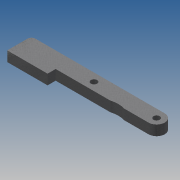
# Autodesk Inventor part: Drückbrücke
Saved by Autodesk Inventor 2015 SP1 (Build 190203100, 203)
## iProperties
Created: 2015-01-28
Part Number: Drückbrücke
Material: ABS-Kunststoff
Document SubType Name: Modeling
Designer: Marc
Density: 1.06 g/cm^3
Appearance: Gehont - dunkelgrau
Mass: 3.36639 g
Surface Area: 19.9083 cm^2
Volume: 3.17584 cm^3
Author: Marc
Autodesk Inventor part; units mm, degrees
ref_plane "YZ Plane" through (0, 0, 0) normal (1, 0, 0) x (0, 1, 0)
ref_plane "XZ Plane" through (0, 0, 0) normal (0, 1, 0) x (-1, 0, 0)
ref_plane "XY Plane" through (0, 0, 0) normal (0, 0, 1) x (1, 0, 0)
sketch "Skizze1" plane through (0, 0, 0) normal (0, 0, 1) x (1, 0, 0)
  line L0 (0, -28.5) -> (0, 27.5) projected
  line L1 (-71.9, 0) -> (35.9, 0) projected
  circle A0 centre (-15.5, 15.5) radius 1.55
  circle A1 centre (15.5, 15.5) radius 1.55
  circle A2 centre (-15.5, -15.5) radius 1.55
  circle A3 centre (15.5, -15.5) radius 1.55
  circle A4 centre (-16.5, 0) radius 11
  circle A5 centre (0, 0) radius 5.5
  circle A6 centre (-16.5, 0) radius 4
  arc A7 (-16.5, -7.5) -> (-16.5, 7.5) centre (-16.5, 0) ccw
  line L2 (-16.5, 7.5) -> (-36.5, 7.5)
  line L3 (-36.5, 7.5) -> (-56.5, 7.5)
  line L4 (-56.5, 7.5) -> (-56.5, -7.5)
  line L5 (-56.5, -7.5) -> (-16.5, -7.5)
  circle A8 centre (15.5, 15.5) radius 4
  circle A9 centre (15.5, -15.5) radius 5
  circle A10 centre (-15.5, 15.5) radius 4
  circle A11 centre (-15.5, -15.5) radius 4
  line L6 (15.5, 11.5) -> (-15.5, 11.5)
  line L7 (15.5, 19.5) -> (-15.5, 19.5)
  line L8 (-15.5, 19.5) -> (-50.5, 19.5)
  line L9 (-50.5, 19.5) -> (-50.5, 7.5)
  line L10 (-15.5, 11.5) -> (-30.5, 11.5)
  line L11 (-30.5, 11.5) -> (-30.5, 7.5)
  dimension "d0" = 3.1
  dimension "d1" = 15.5
  dimension "d2" = 15.5
  dimension "d3" = 22
  dimension "d4" = 16.5
  dimension "d5" = 11
  dimension "d6" = 8
  dimension "d7" = 15
  dimension "d10" = 15
  dimension "d11" = 40
  dimension "d17" = 8
  dimension "d18" = 10
  dimension "d19" = 8
  dimension "d20" = 8
  dimension "d22" = 35
  dimension "d23" = 15
  constraints: 20 end point, 12 centre point, 7 coincident, 6 point on circle, 4 point on line, 4 tangent, 3 horizontal, 3 perpendicular, 3 symmetric about line, 3 other
  measures "d0" diameter of A0
  measures "d1" distance from line of L1 A0.centre
  measures "d2" distance from line of L0 A0.centre
  measures "d3" diameter of A4
  measures "d4" distance from line of L0 A4.centre
  measures "d5" diameter of A5
  measures "d6" diameter of A6
  measures "d7" diameter of A7
  measures "d10" distance of L3.end L4.end
  measures "d11" distance from line of L2.start L4
  measures "d17" diameter of A8
  measures "d18" diameter of A9
  measures "d19" diameter of A10
  measures "d20" diameter of A11
  measures "d22" distance of L7.end L8.end
  measures "d23" distance of L6.end L10.end
extrude "Extrusion3" add sketch "Skizze1" along normal blind 5 contours L6 A10 L7 L0 | L0 L7 A8 L6 | L2 L3 L9 L8 A10 L10 L11 | A8 | A10
sketch "Skizze3" plane through (0, 0, 5) normal (0, 0, 1) x (1, 0, 0)
  circle A0 centre (0, 0) radius 12 projected
  circle A1 centre (-13.5, -33.5) radius 2.75 projected
  circle A2 centre (13.5, -33.5) radius 2.75 projected
  circle A3 centre (-15.5, -15.5) radius 1.75 projected
  circle A4 centre (15.5, -15.5) radius 1.75 projected
  circle A5 centre (-15.5, 15.5) radius 1.75 projected
  circle A6 centre (15.5, 15.5) radius 1.75 projected
  line L0 (19.5, -43.5) -> (21.5, -41.5) projected
  line L1 (21.5, -41.5) -> (21.5, 19.5) projected
  line L2 (21.5, 19.5) -> (19.5, 21.5) projected
  line L3 (19.5, 21.5) -> (-19.5, 21.5) projected
  line L4 (-19.5, 21.5) -> (-21.5, 19.5) projected
  line L5 (-21.5, 19.5) -> (-21.5, -41.5) projected
  line L6 (-21.5, -41.5) -> (-19.5, -43.5) projected
  line L7 (-19.5, -43.5) -> (19.5, -43.5) projected
  line L8 (-30.5, 11.5) -> (15.5, 11.5) projected
  line L9 (3.4278, 11.5) -> (-3.4278, 11.5)
  point P0 (0, 0)
  constraints: 2 end point, 2 point on circle, 2 point on line
extrude "Extrusion4" cut sketch "Skizze3" against normal blind 5 contours L8 A0 picked at (0.3856, 11.648)
fillet "Rundung1" radius 2 1 edges at (-50.5, 19.5, 2.5)
